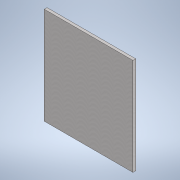
# Autodesk Inventor part: opener_main
Saved by Autodesk Inventor 2021 (Build 250183000, 183)
## iProperties
Created: 2024-04-25
Part Number: opener_main
Material: PC/ABS Plastic
Document SubType Name: Modeling
Designer: ASUS
Density: 0.357273 g/cm^3
Appearance: Weld - Steel Mild
Author: ASUS
Autodesk Inventor part; units mm, degrees
ref_plane "YZ Plane" through (0, 0, 0) normal (1, 0, 0) x (0, 1, 0)
ref_plane "XZ Plane" through (0, 0, 0) normal (0, 1, 0) x (-1, 0, 0)
ref_plane "XY Plane" through (0, 0, 0) normal (0, 0, 1) x (1, 0, 0)
sketch "Sketch1" plane through (0, 0, 0) normal (0, 0, 1) x (1, 0, 0)
  line L0 (0, 0) -> (320, 0)
  line L1 (320, 0) -> (320, 350)
  line L2 (320, 350) -> (0, 350)
  line L3 (0, 350) -> (0, 0)
  dimension "d0" = 320
  dimension "d1" = 350
  constraints: 8 end point, 2 parallel, 1 horizontal, 1 perpendicular
  measures "d0" distance of L2.end L1.end
  measures "d1" distance between parallel lines of L0 L2
extrude "Extrusion1" add sketch "Sketch1" along normal blind 10
body "Solid1"
